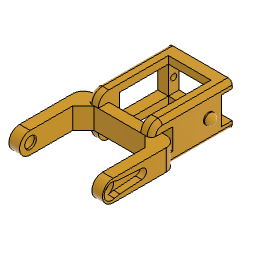
grid_lasercut_plade_assembly v22 (Autodesk Fusion 360 archive; units mm, degrees)
design "link"
Autodesk Fusion 360 part; units mm, degrees
note: some values were not read from the file. Chosen so that the rebuilt part matches the saved one: which bodies a step acts on. Set by a fixed rule: which sketch regions a step uses.
sketch "Sketch1" plane through (0, 0, 0) normal (1, 0, 0) x (0, 1, 0)
  line L0 (0, 0) -> (50, 0)
  line L1 (50, 0) -> (50, 10)
  line L2 (50, 10) -> (0, 10)
  line L3 (0, 10) -> (0, 0)
  dimension "d1" = 50
  dimension "d2" = 10
  constraint horizontal L0
  constraint vertical L1
  constraint horizontal L2
  constraint vertical L3
  constraint coincident L0.start L3.end
  measures "d1" distance of L0.start L0.end
  measures "d2" distance of L0.start L2.end
extrude "Extrude1" add sketch "Sketch1" along normal blind 5 makes body 1
sketch "Sketch2" plane through (5, 0, 0) normal (1, 0, 0) x (0, 1, 0)
  line L0 (0, 10) -> (0, 0)
  line L1 (0, 0) -> (50, 0)
  line L2 (50, 0) -> (50, 10)
  line L3 (50, 10) -> (0, 10)
  line L4 (0, 5) -> (4.5, 5) construction
  circle A0 centre (4.5, 5) radius 3.7
  line L5 (4.5, 5) -> (6.5, 5) construction
  line L6 (6.5, 5) -> (6.5, 8.1129)
  line L7 (6.5, 5) -> (6.5, 1.8871)
  line L8 (4.5, 5) -> (18.5, 5) construction
  circle A1 centre (18.5, 5) radius 2.25
  line L9 (18.5, 5) -> (18.5, 7.25) construction
  line L10 (18.5, 5) -> (18.5, 2.75) construction
  line L11 (6.5, 1.8871) -> (18.5, 2.75)
  line L12 (6.5, 8.1129) -> (18.5, 7.25)
  dimension "d5" = 4.5
  dimension "d6" = 7.4
  dimension "d11" = 2
  dimension "d12" = 14
  dimension "d13" = 4.5
  constraint midpoint L0 L4.start
  constraint perpendicular L0 L4
  constraint coincident L4.end A0.centre
  constraint parallel L4 L5
  constraint coincident A0 L6.end
  constraint perpendicular L5 L6
  constraint coincident A0 L7.end
  constraint perpendicular L5 L7
  constraint parallel L5 L8
  constraint coincident L8.end A1.centre
  constraint coincident A1 L9.end
  constraint perpendicular L8 L9
  constraint coincident A1 L10.end
  constraint perpendicular L8 L10
  measures "d5" distance of L4.start L4.end
  measures "d6" diameter of A0
  measures "d11" distance of L4.end L5.end
  measures "d12" distance of L4.end L8.end
  measures "d13" diameter of A1
extrude "Extrude2" cut sketch "Sketch2" against normal blind 5 contours A0 L6 L7 | A0 L6 L7 bodies 1
fillet "Fillet1" radius 5 2 edges at (2.5, 0, 10) (2.5, 0, 0) on bodies 1
extrude "Extrude3" cut sketch "Sketch2" against normal blind 3 contours A0 A1 L11 L12 | A1 bodies 1
fillet "Fillet2" radius 10 2 edges at (3.5, 6.5, 8.1129) (3.5, 6.5, 1.8871) on bodies 1
sketch "Sketch3" plane through (0, 0, 0) normal (-1, 0, 0) x (0, -1, 0)
  circle A0 centre (-4.5, 5) radius 3.7
  arc A1 (-5, 0) -> (-5, 10) centre (-5, 5) ccw
  line L0 (-5, 10) -> (-50, 10)
  line L1 (-50, 10) -> (-50, 0)
  line L2 (-50, 0) -> (-5, 0)
  line L3 (-50, 10) -> (-30, 10) construction
  line L4 (-30, 10) -> (-30, 0) construction
  line L5 (-30, 0) -> (-50, 0) construction
  line L6 (-50, 0) -> (-50, 10) construction
  line L7 (-30, 10) -> (-35, 10)
  line L8 (-35, 10) -> (-35, 0)
  line L9 (-35, 0) -> (-30, 0)
  line L10 (-30, 0) -> (-30, 10)
  dimension "d18" = 20
  dimension "d19" = 5
  constraint horizontal L3
  constraint vertical L4
  constraint horizontal L5
  constraint vertical L6
  constraint coincident L0.end L1.start
  constraint horizontal L7
  constraint vertical L8
  constraint horizontal L9
  constraint vertical L10
  measures "d18" distance of L0.end L3.end
  measures "d19" distance of L3.end L7.end
extrude "Extrude4" add sketch "Sketch3" along normal blind 39 contours L0 L2 L7 L8 L9 L10 bodies 1
sketch "Sketch4" plane through (0, 30, 0) normal (0, -1, 0) x (1, 0, 0)
  line L0 (0, 0) -> (0, 10)
  line L1 (0, 10) -> (-39, 10)
  line L2 (-39, 10) -> (-39, 0)
  line L3 (-39, 0) -> (0, 0)
  line L4 (-39, 10) -> (-34, 10)
  line L5 (-34, 10) -> (-34, 0)
  line L6 (-34, 0) -> (-39, 0)
  line L7 (-39, 0) -> (-39, 10)
  dimension "d22" = 5
  constraint horizontal L4
  constraint vertical L5
  constraint horizontal L6
  constraint vertical L7
  constraint coincident L1.end L2.start
  measures "d22" distance of L1.end L4.end
extrude "Extrude5" add sketch "Sketch4" along normal blind 30 contours L1 L2 L3 L4 L5 L6 L7 bodies 1
sketch "Sketch5" plane through (-34, 0, 0) normal (1, 0, 0) x (0, 1, 0)
  line L0 (30, 0) -> (30, 10)
  line L1 (30, 10) -> (0, 10)
  line L2 (0, 10) -> (0, 0)
  line L3 (0, 0) -> (30, 0)
  line L4 (0, 5) -> (5.175, 5) construction
  circle A0 centre (5.175, 5) radius 2.75
  dimension "d25" = 5.175
  dimension "d26" = 5.5
  constraint midpoint L2 L4.start
  constraint perpendicular L2 L4
  constraint coincident L4.end A0.centre
  measures "d25" distance of L4.start L4.end
  measures "d26" diameter of A0
extrude "Extrude6" cut sketch "Sketch5" against normal blind 3 contours A0 bodies 1
fillet "Fillet3" radius 2 1 edges at (-37, 2.6111, 5.9944) on bodies 1
fillet "Fillet4" radius 5 2 edges at (-36.5, 0, 10) (-36.5, 0, 0) on bodies 1
extrude "Extrude7" cut 1 faces at (1.6667, 50, 3.3333) along direction (0, -1, 0) blind 10 on bodies 1 bodies 1
sketch "Sketch6" plane through (0, 0, 0) normal (0, 0, -1) x (1, 0, 0)
  line L0 (0, -40) -> (5, -40)
  line L1 (5, -40) -> (5, -5)
  line L2 (5, -5) -> (0, -5)
  line L3 (0, -5) -> (0, -30)
  line L4 (0, -30) -> (-34, -30)
  line L5 (-34, -30) -> (-34, -5)
  line L6 (-34, -5) -> (-39, -5)
  line L7 (-39, -5) -> (-39, -35)
  line L8 (-39, -35) -> (0, -35)
  line L9 (0, -35) -> (0, -40)
  line L10 (0, -40) -> (5, -40)
  line L11 (5, -40) -> (5, -35)
  line L12 (5, -35) -> (0, -35)
  line L13 (0, -35) -> (0, -40)
  dimension "d35" = 5
  constraint horizontal L10
  constraint vertical L11
  constraint horizontal L12
  constraint vertical L13
  constraint coincident L0.start L9.end
  measures "d35" distance of L0.start L8.end
extrude "Extrude8" add sketch "Sketch6" along normal blind 5 contours L0 L1 L9 L10 L11 L12 L13 bodies 1
sketch "Sketch7" plane through (0, 0, 10) normal (0, 0, 1) x (-1, 0, 0)
  line L0 (-5, -40) -> (0, -40)
  line L1 (0, -40) -> (0, -35)
  line L2 (0, -35) -> (39, -35)
  line L3 (39, -35) -> (39, -5)
  line L4 (39, -5) -> (34, -5)
  line L5 (34, -5) -> (34, -30)
  line L6 (34, -30) -> (0, -30)
  line L7 (0, -30) -> (0, -5)
  line L8 (0, -5) -> (-5, -5)
  line L9 (-5, -5) -> (-5, -40)
  line L10 (0, -40) -> (-5, -40)
  line L11 (-5, -40) -> (-5, -35)
  line L12 (-5, -35) -> (0, -35)
  line L13 (0, -35) -> (0, -40)
  dimension "d38" = 5
  constraint horizontal L10
  constraint vertical L11
  constraint horizontal L12
  constraint vertical L13
  constraint coincident L0.end L1.start
  measures "d38" distance of L0.end L1.end
extrude "Extrude9" add sketch "Sketch7" along normal blind 5 contours L0 L1 L9 L10 L11 L12 L13 bodies 1
sketch "Sketch8" plane through (0, 35, 0) normal (0, 1, 0) x (-1, 0, 0)
  line L0 (0, 10) -> (0, 0)
  line L1 (0, 0) -> (39, 0)
  line L2 (39, 0) -> (39, 10)
  line L3 (39, 10) -> (0, 10)
  line L4 (39, 0) -> (34, 0)
  line L5 (34, 0) -> (34, 15)
  line L6 (34, 15) -> (39, 15)
  line L7 (39, 15) -> (39, 0)
  line L8 (39, 0) -> (34, 0)
  line L9 (34, 0) -> (34, -5)
  line L10 (34, -5) -> (39, -5)
  line L11 (39, -5) -> (39, 0)
  dimension "d41" = 5
  dimension "d42" = 15
  dimension "d43" = 5
  dimension "d44" = 5
  constraint horizontal L4
  constraint vertical L5
  constraint horizontal L6
  constraint vertical L7
  constraint coincident L1.end L2.start
  constraint horizontal L8
  constraint vertical L9
  constraint horizontal L10
  constraint vertical L11
  measures "d41" distance of L1.end L4.end
  measures "d42" distance of L1.end L6.end
  measures "d43" distance of L1.end L4.end
  measures "d44" distance of L1.end L10.end
extrude "Extrude10" add sketch "Sketch8" along normal blind 5 contours L3 L5 L6 L7 | L1 L2 L3 L4 L5 L7 L8 | L1 L4 L8 L9 L10 L11 bodies 1
split "Split1" by plane through (0, 35, 10) normal (0, 1, 0) bodies 1 makes body 2 at (-39, 38.3333, 3.3333) makes body 3 at (5, 38.3333, 6.6667)
move_body "Move1" bodies 2 to x (1, 0, 0) y (0, 1, 0) z (0, 0, 1) at (7, 0, 0)
move_body "Move2" bodies 3 to x (1, 0, 0) y (0, 1, 0) z (0, 0, 1) at (-7, 0, 0)
combine "Combine1" operation add target body 2 tool bodies 3 1
revolve "Revolve1" add 2 faces at (-28.6667, 35, -1.6667) (-3.6667, 35, -1.6667) angle 360 about axis through (-27, 35, 0) along (1, 0, 0) on bodies 2 bodies 2
revolve "Revolve2" add 2 faces at (-30.3333, 35, 11.6667) (-3.6667, 35, 11.6667) angle 360 about axis through (-7, 35, 10) along (-1, 0, 0) on bodies 2 bodies 2
sketch "Sketch9" plane through (-27, 0, 0) normal (1, 0, 0) x (0, 1, 0)
  arc A0 (30, 0) -> (35, -5) centre (35, 0) ccw
  line L0 (35, -5) -> (40, -5)
  line L1 (40, -5) -> (40, 15)
  line L2 (40, 15) -> (35, 15)
  arc A1 (35, 15) -> (30, 10) centre (35, 10) ccw
  line L3 (35, 5) -> (37.6, 5) construction
  circle A2 centre (37.6, 5) radius 1.4
  line L4 (30, 10) -> (35, 10)
  line L5 (35, 10) -> (35, 0)
  line L6 (35, 0) -> (30, 0)
  dimension "d49" = 2.6
  dimension "d50" = 2.8
  constraint coincident L3.end A2.centre
  measures "d49" distance of L3.start L3.end
  measures "d50" diameter of A2
extrude "Extrude11" cut sketch "Sketch9" against normal blind 5 contours A2 bodies 2
sketch "Sketch10" plane through (0, 40, 0) normal (0, 1, 0) x (-1, 0, 0)
  line L0 (27, 15) -> (27, -5)
  line L1 (27, -5) -> (32, -5)
  line L2 (32, -5) -> (32, 15)
  line L3 (32, 15) -> (27, 15)
  line L4 (27, -5) -> (39, -5)
  line L5 (39, -5) -> (39, -1.5)
  line L6 (39, -1.5) -> (27, -1.5)
  line L7 (27, -1.5) -> (27, -5)
  line L8 (27, 15) -> (39, 15)
  line L9 (39, 15) -> (39, 11.5)
  line L10 (39, 11.5) -> (27, 11.5)
  line L11 (27, 11.5) -> (27, 15)
  dimension "d57" = 3.5
  dimension "d58" = 3.5
  constraint horizontal L4
  constraint vertical L5
  constraint horizontal L6
  constraint vertical L7
  constraint coincident L0.end L1.start
  constraint horizontal L8
  constraint vertical L9
  constraint horizontal L10
  constraint vertical L11
  constraint coincident L0.start L3.end
  measures "d57" distance of L0.end L6.end
  measures "d58" distance of L0.start L10.end
extrude "Extrude12" add sketch "Sketch10" along normal blind 28 contours L0 L2 L3 L8 L10 L11 | L0 L1 L2 L4 L6 L7 bodies 2
sketch "Sketch11" plane through (0, 0, 11.5) normal (0, 0, -1) x (1, 0, 0)
  line L0 (-27, -40) -> (-32, -40)
  line L1 (-32, -40) -> (-32, -68)
  line L2 (-32, -68) -> (-27, -68)
  line L3 (-27, -68) -> (-27, -40)
  line L4 (-27, -68) -> (-32, -68)
  line L5 (-32, -68) -> (-32, -63)
  line L6 (-32, -63) -> (-27, -63)
  line L7 (-27, -63) -> (-27, -68)
  dimension "d61" = 5
  constraint horizontal L4
  constraint vertical L5
  constraint horizontal L6
  constraint vertical L7
  constraint coincident L2.end L3.start
  measures "d61" distance of L2.end L6.end
extrude "Extrude13" add sketch "Sketch11" along normal blind 13 contours L1 L2 L3 L4 L5 L6 L7 bodies 2
sketch "Sketch12" plane through (-32, 0, 0) normal (-1, 0, 0) x (0, -1, 0)
  line L0 (-63, 11.5) -> (-40, 11.5)
  line L1 (-40, 11.5) -> (-40, -1.5)
  line L2 (-40, -1.5) -> (-63, -1.5)
  line L3 (-63, -1.5) -> (-63, 11.5)
  circle A0 centre (-37.6, 5) radius 1.4
  line L4 (-68, 15) -> (-68, -5)
  line L5 (-68, -5) -> (-35, -5)
  arc A1 (-35, -5) -> (-30, 0) centre (-35, 0) ccw
  arc A2 (-30, 10) -> (-35, 15) centre (-35, 10) ccw
  line L6 (-35, 15) -> (-68, 15)
  line L7 (-63, 5) -> (-65.5, 5) construction
  circle A3 centre (-65.5, 5) radius 1.4
  line L8 (-30, 0) -> (-35, 0)
  line L9 (-35, 0) -> (-35, 10)
  line L10 (-35, 10) -> (-30, 10)
  dimension "d64" = 2.5
  dimension "d65" = 2.8
  constraint midpoint L3 L7.start
  constraint perpendicular L4 L7
  constraint coincident L7.end A3.centre
  measures "d64" distance of L7.start L7.end
  measures "d65" diameter of A3
extrude "Extrude14" cut sketch "Sketch12" against normal blind 5 contours A3 bodies 2
extrude "Extrude15" add 1 faces at (-5.3333, 40, 8.3333) along direction (0, 1, 0) blind 28 on bodies 2 bodies 2
chamfer "Chamfer1" distance 5 angle 45 2 edges at (0, 30, 5) (-34, 30, 5) on bodies 2
fillet "Fillet5" radius 5 2 edges at (5, 35, 5) (-39, 35, 5) on bodies 2
sketch "Sketch13" plane through (-27, 0, 0) normal (1, 0, 0) x (0, 1, 0)
  circle A0 centre (65.5, 5) radius 1.4
  line L0 (68, -5) -> (68, 15)
  line L1 (68, 15) -> (35, 15)
  arc A1 (35, 15) -> (30, 10) centre (35, 10) ccw
  line L2 (30, 10) -> (35, 10)
  line L3 (35, 10) -> (35, 0)
  line L4 (35, 0) -> (30, 0)
  arc A2 (30, 0) -> (35, -5) centre (35, 0) ccw
  line L5 (35, -5) -> (68, -5)
  circle A3 centre (37.6, 5) radius 1.4
  line L6 (63, 11.5) -> (63, -1.5)
  line L7 (63, -1.5) -> (40, -1.5)
  line L8 (40, -1.5) -> (40, 11.5)
  line L9 (40, 11.5) -> (63, 11.5)
  line L10 (68, 15) -> (63, 15)
  line L11 (63, 15) -> (63, 11.5)
  line L12 (63, 11.5) -> (68, 11.5)
  line L13 (68, 11.5) -> (68, 15)
  line L14 (68, -5) -> (63, -5)
  line L15 (63, -5) -> (63, -1.5)
  line L16 (63, -1.5) -> (68, -1.5)
  line L17 (68, -1.5) -> (68, -5)
  constraint horizontal L10
  constraint vertical L11
  constraint horizontal L12
  constraint vertical L13
  constraint coincident L6.start L9.end
  constraint coincident L0.end L1.start
  constraint horizontal L14
  constraint vertical L15
  constraint horizontal L16
  constraint vertical L17
  constraint coincident L6.end L7.start
  constraint coincident L0.start L5.end
extrude "Extrude16" add sketch "Sketch13" along normal blind 20 contours L0 L5 L14 L15 L16 L17 | L0 L1 L10 L11 L12 L13 bodies 2
sketch "Sketch14" plane through (-2, 0, 0) normal (1, 0, 0) x (0, 1, 0)
  line L0 (35, 10) -> (35, 0)
  line L1 (35, 0) -> (30, 0)
  arc A0 (30, 0) -> (35, -5) centre (35, 0) ccw
  line L2 (35, -5) -> (68, -5)
  line L3 (68, -5) -> (68, 15)
  line L4 (68, 15) -> (35, 15)
  arc A1 (35, 15) -> (30, 10) centre (35, 10) ccw
  line L5 (30, 10) -> (35, 10)
  line L6 (68, 15) -> (68, 11.5) construction
  line L7 (68, 11.5) -> (63, 11.5)
  line L8 (63, 11.5) -> (63, -1.5)
  line L9 (63, -1.5) -> (68, -1.5)
  line L10 (68, -1.5) -> (68, 11.5)
  line L11 (35, 10) -> (40, 10)
  line L12 (40, 10) -> (40, 0)
  line L13 (40, 0) -> (35, 0)
  line L14 (35, 0) -> (35, 10)
  dimension "d75" = 3.5
  dimension "d76" = 5
  dimension "d77" = 13
  dimension "d80" = 5
  dimension "d81" = 10
  constraint coincident L3.end L4.start
  constraint perpendicular L2 L6
  constraint horizontal L7
  constraint vertical L8
  constraint horizontal L9
  constraint vertical L10
  constraint horizontal L11
  constraint vertical L12
  constraint horizontal L13
  constraint vertical L14
  constraint coincident L0.start A1.centre
  measures "d75" distance of L3.end L6.end
  measures "d76" distance of L6.end L7.end
  measures "d77" distance of L6.end L9.end
  measures "d80" distance of L0.start L11.end
  measures "d81" distance of L0.start L0.end
extrude "Extrude17" cut sketch "Sketch14" against normal blind 5 contours L0 L11 L12 L13 L14 | L3 L7 L8 L9 L10 bodies 2
fillet "Fillet6" radius 2 8 edges at (-32, 31.4645, 13.5355) (-32, 51.5, 15) (-2, 31.4645, 13.5355) (-2, 51.5, 15) (-2, 31.4645, -3.5355) (-2, 51.5, -5) (-32, 31.4645, -3.5355) (-32, 51.5, -5) on bodies 2
sketch "Sketch15" plane through (-2, 0, 0) normal (1, 0, 0) x (0, 1, 0)
  arc A0 (32, 0) -> (35, -3) centre (35, 0) ccw
  line L0 (35, -3) -> (68, -3)
  line L1 (68, -3) -> (68, -1.5)
  line L2 (68, -1.5) -> (63, -1.5)
  line L3 (63, -1.5) -> (63, 11.5)
  line L4 (63, 11.5) -> (68, 11.5)
  line L5 (68, 11.5) -> (68, 13)
  line L6 (68, 13) -> (35, 13)
  arc A1 (35, 13) -> (32, 10) centre (35, 10) ccw
  line L7 (32, 10) -> (35, 10)
  line L8 (35, 10) -> (40, 10)
  line L9 (40, 10) -> (40, 0)
  line L10 (40, 0) -> (35, 0)
  line L11 (35, 0) -> (32, 0)
  line L12 (63, 5) -> (57, 5) construction
  circle A2 centre (57, 5) radius 2.5
  dimension "d84" = 6
  dimension "d85" = 5
  constraint midpoint L3 L12.start
  constraint perpendicular L9 L12
  constraint coincident L12.end A2.centre
  measures "d84" distance of L12.start L12.end
  measures "d85" diameter of A2
extrude "Extrude18" add sketch "Sketch15" along normal blind 3 contours A2 bodies 2
fillet "Fillet7" radius 2.5 1 edges at (1, 54.6692, 4.096) on bodies 2

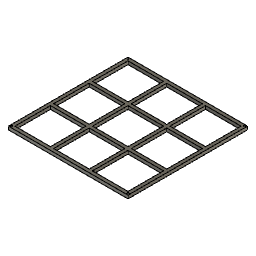
design "Play_board"
Autodesk Fusion 360 part; units mm, degrees
sketch "Sketch1" plane through (0, 0, 0) normal (0, 0, 1) x (1, 0, 0)
  line L0 (110, -92.5) -> (-110, -92.5)
  line L1 (-110, -92.5) -> (-110, 92.5)
  line L2 (-110, 92.5) -> (110, 92.5)
  line L3 (110, 92.5) -> (110, -92.5)
  line L4 (110, -92.5) -> (-110, 92.5) construction
  line L5 (-110, -92.5) -> (110, 92.5) construction
  line L6 (-110, 92.5) -> (97.5144, 92.5)
  line L7 (-53.7181, -92.5) -> (-110, -92.5)
  line L8 (-110, -92.5) -> (-110, 92.5)
  line L9 (-50, 92.5) -> (-45, 92.5)
  line L10 (-45, 92.5) -> (-45, -92.5)
  line L11 (-45, -92.5) -> (-50, -92.5)
  line L12 (-50, -92.5) -> (-50, 92.5)
  line L13 (10, 92.5) -> (15, 92.5)
  line L14 (15, 92.5) -> (15, -92.5)
  line L15 (15, -92.5) -> (10, -92.5)
  line L16 (10, -92.5) -> (10, 92.5)
  line L17 (70, 92.5) -> (75, 92.5)
  line L18 (75, 92.5) -> (75, -92.5)
  line L19 (75, -92.5) -> (70, -92.5)
  line L20 (70, -92.5) -> (70, 92.5)
  line L21 (75, 42.0875) -> (75, 63.0682)
  line L22 (-110, 68) -> (-110, 42.0875)
  line L23 (75, -17.4811) -> (75, -23.4712)
  line L24 (-110, -23.4712) -> (-110, -17.4811)
  line L25 (-110, 32.5) -> (75, 32.5)
  line L26 (75, 32.5) -> (75, 27.5)
  line L27 (75, 27.5) -> (-110, 27.5)
  line L28 (-110, 27.5) -> (-110, 32.5)
  line L29 (-110, -27.5) -> (75, -27.5)
  line L30 (75, -27.5) -> (75, -32.5)
  line L31 (75, -32.5) -> (-110, -32.5)
  line L32 (-110, -32.5) -> (-110, -27.5)
  line L33 (-110, -87.5) -> (75, -87.5)
  line L34 (75, -87.5) -> (75, -92.5)
  line L35 (75, -92.5) -> (-110, -92.5)
  line L36 (-110, -92.5) -> (-110, -87.5)
  line L37 (-110, 92.5) -> (75, 92.5)
  line L38 (75, 92.5) -> (75, 87.5)
  line L39 (75, 87.5) -> (-110, 87.5)
  line L40 (-110, 87.5) -> (-110, 92.5)
  line L41 (-110, 92.5) -> (-105, 92.5)
  line L42 (-105, 92.5) -> (-105, -92.5)
  line L43 (-105, -92.5) -> (-110, -92.5)
  line L44 (-110, -92.5) -> (-110, 92.5)
  line L45 (75, 37.5) -> (110, 37.5) construction
  line L46 (75, -37.5) -> (110, -37.5) construction
  circle A0 centre (76.8705, -4.3263) radius 25 construction
  circle A1 centre (78.6242, -22.2407) radius 1.75
  circle A2 centre (76.6017, 13.6717) radius 1.75
  line L47 (75, 25.3235) -> (110, 25.3235) construction
  dimension "d3" = 220
  dimension "d5" = 5
  dimension "d6" = 5
  dimension "d8" = 5
  dimension "d10" = 55
  dimension "d11" = 55
  dimension "d13" = 5
  dimension "d16" = 5
  dimension "d17" = 5
  dimension "d18" = 5
  dimension "d19" = 55
  dimension "d20" = 55
  dimension "d22" = 55
  dimension "d23" = 5
  dimension "d24" = 55
  dimension "d25" = 55
  dimension "d26" = 55
  dimension "d27" = 50
  dimension "d32" = 3.5
  dimension "d33" = 3.5
  dimension "d34" = 18
  dimension "d35" = 18
  constraint horizontal L0
  constraint perpendicular L0 L1
  constraint parallel L0 L2
  constraint parallel L1 L3
  constraint coincident L4 origin
  constraint coincident L5 origin
  constraint horizontal L6
  constraint horizontal L7
  constraint vertical L8
  constraint coincident L0 L7.start
  constraint horizontal L9
  constraint vertical L10
  constraint horizontal L11
  constraint vertical L12
  constraint coincident L0 L10.end
  constraint coincident L2 L9.start
  constraint horizontal L13
  constraint vertical L14
  constraint horizontal L15
  constraint vertical L16
  constraint coincident L0 L14.end
  constraint coincident L2 L13.start
  constraint horizontal L17
  constraint vertical L18
  constraint horizontal L19
  constraint vertical L20
  constraint coincident L0 L18.end
  constraint coincident L2 L17.start
  constraint vertical L21
  constraint vertical L22
  constraint coincident L18 L21.end
  constraint coincident L5 L21.end
  constraint coincident L8 L22.end
  constraint vertical L23
  constraint vertical L24
  constraint coincident L18 L23.end
  constraint coincident L1 L24.end
  constraint horizontal L25
  constraint vertical L26
  constraint horizontal L27
  constraint vertical L28
  constraint coincident L18 L26.end
  constraint coincident L8 L25.start
  constraint horizontal L29
  constraint vertical L30
  constraint horizontal L31
  constraint vertical L32
  constraint coincident L18 L30.end
  constraint coincident L1 L29.start
  constraint horizontal L33
  constraint vertical L34
  constraint horizontal L35
  constraint vertical L36
  constraint coincident L8 L33.start
  constraint horizontal L37
  constraint vertical L38
  constraint horizontal L39
  constraint vertical L40
  constraint coincident L18 L38.end
  constraint horizontal L41
  constraint vertical L42
  constraint horizontal L43
  constraint vertical L44
  constraint coincident L7 L42.end
  constraint coincident L18 L45.start
  constraint coincident L3 L45.end
  constraint perpendicular L3 L45
  constraint coincident L18 L46.start
  constraint coincident L3 L46.end
  constraint perpendicular L3 L46
  constraint coincident L18 L47.start
  constraint coincident L3 L47.end
  constraint perpendicular L3 L47
  measures "d3" distance of L1.end L2.end
  measures "d5" distance of L10 L12
  measures "d6" distance of L14 L16
  measures "d8" distance of L18 L20
  measures "d10" distance of L10 L16
  measures "d11" distance of L14 L20
  measures "d13" distance of L25 L27
  measures "d16" distance of L29 L31
  measures "d17" distance of L0 L33
  measures "d18" distance of L2 L39
  measures "d19" distance of L25 L39
  measures "d20" distance of L27 L29
  measures "d22" distance of L31 L33
  measures "d23" distance of L1 L42
  measures "d24" distance of L12 L42
  measures "d25" distance of L2 L45
  measures "d26" distance of L0 L46
  measures "d27" diameter of A0
  measures "d32" diameter of A1
  measures "d33" diameter of A2
  measures "d34" distance of A0.centre A2.centre
  measures "d35" distance of A0.centre A1.centre
extrude "Extrude7" add sketch "Sketch1" along normal blind 5 contours L0 L18 L19 L20 L33 L34 L35 | L0 L14 L20 L33 L35 | L18 L20 L31 L33 | L0 L14 L15 L16 L33 L35 | L18 L20 L29 L30 L31 | L2 L6 L17 L18 L20 L37 L38 L39 | L0 L10 L16 L33 L35 | L14 L16 L31 L33 | L14 L20 L29 L31 | L18 L20 L23 L27 L29 A2 | L2 L6 L14 L20 L37 L39 | L18 L20 L21 L25 L39 | L0 L10 L11 L12 L33 L35 | L14 L16 L29 L31 | L2 L6 L13 L14 L16 L37 L39 | L0 L7 L12 L33 L35 L42 | L10 L12 L31 L33 | L10 L16 L29 L31 | L14 L16 L27 L29 | L14 L20 L25 L27 | L18 L20 L25 L26 L27 | L2 L6 L10 L16 L37 L39 | L14 L16 L25 L39 | L10 L12 L29 L31 | L14 L16 L25 L27 | L18 A2 | L2 L6 L9 L10 L12 L37 L39 | L0 L1 L7 L8 L33 L35 L36 L42 L43 L44 | L12 L29 L31 L42 | L1 L8 L31 L33 L42 L44 | L10 L12 L27 L29 | L10 L16 L25 L27 | L2 L6 L12 L37 L39 L42 | L10 L12 L25 L39 | L1 L8 L29 L31 L32 L42 L44 | L10 L12 L25 L27 | L1 L2 L6 L8 L37 L39 L40 L41 L42 L44 | L12 L25 L27 L42 | L1 L8 L24 L27 L29 L42 L44 | L1 L8 L22 L25 L39 L42 L44 | L1 L8 L25 L27 L28 L42 L44 picked at (74.9727, 13.8309)
sketch "Sketch5" plane through (0, 0, 0) normal (0, 0, 1) x (1, 0, 0)
  line L0 (-110, 92.5) -> (-105, 87.5) construction
  line L1 (-105, 92.5) -> (-110, 87.5) construction
  circle A0 centre (-107.5, 90) radius 1.4
  line L2 (70, 92.5) -> (75, 87.5) construction
  line L3 (75, 92.5) -> (70, 87.5) construction
  circle A1 centre (72.5, 90) radius 1.4
  line L4 (70, -87.5) -> (75, -92.5) construction
  line L5 (75, -87.5) -> (70, -92.5) construction
  circle A2 centre (72.5, -90) radius 1.4
  line L6 (-110, -87.5) -> (-105, -92.5) construction
  line L7 (-105, -87.5) -> (-110, -92.5) construction
  circle A3 centre (-107.5, -90) radius 1.4
  dimension "d54" = 2.8
  dimension "d55" = 2.8
  dimension "d56" = 2.8
  dimension "d57" = 2.8
  constraint midpoint L1 A0.centre
  constraint perpendicular L2 L3
  constraint midpoint L3 A1.centre
  constraint midpoint L5 A2.centre
  constraint midpoint L7 A3.centre
  measures "d54" diameter of A0
  measures "d55" diameter of A1
  measures "d56" diameter of A2
  measures "d57" diameter of A3
extrude "Extrude8" cut sketch "Sketch5" along normal through all
equation "Board_piece_lenght = 40 mm"
equation "d5 = Wall_width"
equation "d6 = Wall_width"
equation "Wall_width = 5 mm"
equation "d8 = Wall_width"
equation "d10 = Inner_sqauare"
equation "d11 = Inner_sqauare"
equation "Inner_sqauare = 55 mm"
equation "d13 = Wall_width"
equation "d16 = Wall_width"
equation "d17 = Wall_width"
equation "d18 = Wall_width"
equation "d19 = Inner_sqauare"
equation "d20 = Inner_sqauare"
equation "d22 = Inner_sqauare"
equation "d23 = Wall_width"
equation "d24 = Inner_sqauare"
equation "d25 = Inner_sqauare"
equation "d26 = Inner_sqauare"
